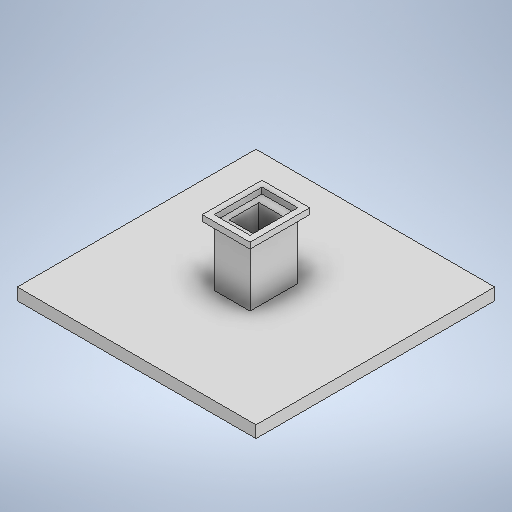
# Autodesk Inventor part: 單線圈感測器
Saved by Autodesk Inventor 2025.2 (Build 292293000, 293)
## iProperties
Created: 2025-06-16
Part Number: 單線圈感測器
Material: 一般
Document SubType Name: Modeling
Designer: 123
Density: 1 g/cm^3
Appearance: 預設
Author: 123
Autodesk Inventor part; units mm, degrees
ref_plane "YZ Plane" through (0, 0, 0) normal (1, 0, 0) x (0, 1, 0)
ref_plane "XZ Plane" through (0, 0, 0) normal (0, 1, 0) x (-1, 0, 0)
ref_plane "XY Plane" through (0, 0, 0) normal (0, 0, 1) x (1, 0, 0)
sketch "草圖1" plane through (0, 0, 0) normal (0, 1, 0) x (-1, 0, 0)
  line L0 (10, 10) -> (-10, 10)
  line L1 (-10, 10) -> (-10, -10)
  line L2 (-10, -10) -> (10, -10)
  line L3 (10, -10) -> (10, 10)
  line L4 (10, 10) -> (-10, -10) construction
  line L5 (-10, 10) -> (10, -10) construction
  point P0 (0, 0)
  dimension "d0" = 20
  dimension "d1" = 20
  constraints: 12 end point, 2 midpoint, 2 parallel, 1 horizontal, 1 perpendicular
  measures "d0" distance of L0.start L0.end
  measures "d1" distance of L2.end L0.start
extrude "擠出1" add sketch "草圖1" along normal blind 1
sketch "草圖2" plane through (0, 1, 0) normal (0, 1, 0) x (1, 0, 0)
  circle A0 centre (0, 0) radius 1
  line L0 (-1.5, 2) -> (1.5, 2)
  line L1 (1.5, 2) -> (1.5, -2)
  line L2 (1.5, -2) -> (-1.5, -2)
  line L3 (-1.5, -2) -> (-1.5, 2)
  line L4 (-1.5, 2) -> (1.5, -2) construction
  line L5 (1.5, 2) -> (-1.5, -2) construction
  dimension "d4" = 2
  dimension "d5" = 4
  dimension "d6" = 3
  constraints: 12 end point, 2 midpoint, 2 parallel, 1 centre point, 1 coincident, 1 horizontal, 1 perpendicular
  measures "d4" diameter of A0
  measures "d5" distance of L0.end L1.end
  measures "d6" distance of L1.end L2.end
extrude "擠出2" add sketch "草圖2" along normal blind 5 contours A0 | L0 L1 L2 L3
sketch "草圖3" plane through (0, 6, 0) normal (0, 1, 0) x (1, 0, 0)
  line L0 (-1, -1.25) -> (1, -1.25)
  line L1 (1, -1.25) -> (1, 1.25)
  line L2 (1, 1.25) -> (-1, 1.25)
  line L3 (-1, 1.25) -> (-1, -1.25)
  line L4 (-1, -1.25) -> (1, 1.25) construction
  line L5 (1, -1.25) -> (-1, 1.25) construction
  point P0 (0, 0)
  dimension "d9" = 2.5
  dimension "d10" = 2
  constraints: 12 end point, 2 midpoint, 2 parallel, 1 horizontal, 1 perpendicular
  measures "d9" distance of L2.end L0.start
  measures "d10" distance of L1.end L2.end
extrude "擠出3" cut sketch "草圖3" against normal blind 5
sketch "草圖4" plane through (0, 6, 0) normal (0, 1, 0) x (1, 0, 0)
  line L0 (-2, 2.5) -> (2, 2.5)
  line L1 (2, 2.5) -> (2, -2.5)
  line L2 (2, -2.5) -> (-2, -2.5)
  line L3 (-2, -2.5) -> (-2, 2.5)
  line L4 (-2, 2.5) -> (2, -2.5) construction
  line L5 (2, 2.5) -> (-2, -2.5) construction
  point P0 (0, 0)
  dimension "d13" = 4
  dimension "d14" = 5
  constraints: 12 end point, 2 midpoint, 2 parallel, 1 horizontal, 1 perpendicular
  measures "d13" distance of L0.start L0.end
  measures "d14" distance of L0.end L1.end
extrude "擠出4" add sketch "草圖4" along normal blind 0.5
sketch "草圖5" plane through (0, 6.5, 0) normal (0, 1, 0) x (1, 0, 0)
  line L0 (1.5, 2) -> (1.5, -2) projected
  line L1 (-1.5, 2) -> (1.5, 2)
  line L2 (1.5, 2) -> (1.5, -2)
  line L3 (1.5, -2) -> (-1.5, -2)
  line L4 (-1.5, -2) -> (-1.5, 2)
  line L5 (-1.5, 2) -> (1.5, -2) construction
  line L6 (1.5, 2) -> (-1.5, -2) construction
  point P0 (0, 0)
  constraints: 12 end point, 2 midpoint, 2 parallel, 1 horizontal, 1 perpendicular
extrude "擠出5" cut sketch "草圖5" against normal blind 0.5
